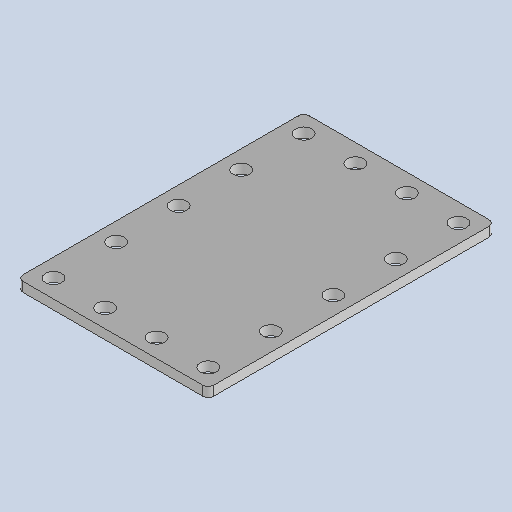
# Autodesk Inventor part: PRS 1607 charging flange rect_940
Saved by Autodesk Inventor 2026.2 (Build 302298000, 298)
## iProperties
Created: 2025-02-13
Part Number: PRS 1607 charging flange rect_940
Material: Steel
Document SubType Name: Sheet Metal
Designer: admin
Mass: 2466.79 g
Surface Area: 934.137 cm^2
Volume: 314.241 cm^3
Density: 7.85 g/cm^3
Flat Pattern Width: 30 cm
Flat Pattern Length: 20 cm
Flat Pattern Area: 600 cm^2
Sheet Metal Rule: AISI304 4mm Die 32
Sheet Metal Width: 300,000 mm
Sheet Metal Length: 200,000 mm
Sheet Metal Area: 60000,000 mm^2
Appearance: Default
Author: pokla
Autodesk Inventor part; units mm, degrees
ref_plane "YZ Plane" through (0, 0, 0) normal (1, 0, 0) x (0, 1, 0)
ref_plane "XZ Plane" through (0, 0, 0) normal (0, 1, 0) x (-1, 0, 0)
ref_plane "XY Plane" through (0, 0, 0) normal (0, 0, 1) x (1, 0, 0)
sketch "Sketch2" plane through (0, 0, 0) normal (0, 0, 1) x (1, 0, 0)
  line L0 (-50, -100) -> (50, -100)
  line L1 (50, -100) -> (50, 100)
  line L2 (50, 100) -> (-50, 100)
  line L3 (-50, 100) -> (-50, -100)
  line L4 (-50, -100) -> (50, 100) construction
  line L5 (50, -100) -> (-50, 100) construction
  line L6 (-100, -150) -> (100, -150)
  line L7 (100, -150) -> (100, 150)
  line L8 (100, 150) -> (-100, 150)
  line L9 (-100, 150) -> (-100, -150)
  point P0 (0, 0)
  dimension "d29" = 100
  dimension "d30" = 200
  dimension "d31" = 50
  measures "d29" distance of L2.end L1.end
  measures "d30" distance of L1.end L0.end
  measures "d31" distance between parallel lines of L3 L9
extrude "Plate2" add sketch "Sketch2" along normal blind 10 contours L3 L2 L1 L0 | L9 L8 L7 L6
sketch "Sketch5" plane through (0, 0, 10) normal (0, 0, 1) x (1, 0, 0)
  line L0 (100, -150) -> (-100, -150) construction
  line L1 (100, 150) -> (100, -150) construction
  line L2 (-100, 150) -> (100, 150) construction
  line L3 (-100, -150) -> (-100, 150) construction
  line L4 (-81, 131) -> (81, 131) construction
  line L5 (81, 131) -> (81, -131) construction
  line L6 (81, -131) -> (-81, -131) construction
  line L7 (-81, -131) -> (-81, 131) construction
  circle A0 centre (-81, -131) radius 8.5
  circle A1 centre (-81, 131) radius 8.5
  circle A2 centre (-81, 0) radius 8.5
  circle A3 centre (-81, -65.5) radius 8.5
  circle A4 centre (-81, 65.5) radius 8.5
  line L8 (-50, 0) -> (50, 0) construction
  circle A5 centre (-27, -131) radius 8.5
  circle A6 centre (-27, -65.5) radius 8.5
  circle A7 centre (-27, 0) radius 8.5
  circle A8 centre (-27, 65.5) radius 8.5
  circle A9 centre (-27, 131) radius 8.5
  circle A10 centre (27, -131) radius 8.5
  circle A11 centre (27, -65.5) radius 8.5
  circle A12 centre (27, 0) radius 8.5
  circle A13 centre (27, 65.5) radius 8.5
  circle A14 centre (27, 131) radius 8.5
  circle A15 centre (81, -131) radius 8.5
  circle A16 centre (81, -65.5) radius 8.5
  circle A17 centre (81, 0) radius 8.5
  circle A18 centre (81, 65.5) radius 8.5
  circle A19 centre (81, 131) radius 8.5
  point P0 (0, 0)
  point P1 (0, -131)
  dimension "d33" = 17
  dimension "d34" = 19
  dimension "d35" = 65.5
  dimension "d36" = 65.5
  dimension "d39" = 54
  constraints: 20 centre point, 10 end point, 8 coincident, 4 equal radius, 2 midpoint, 2 point on line, 1 horizontal, 40 other
  measures "d33" diameter of A0
  measures "d34" distance between parallel lines of L0 L6
  measures "d35" distance of A3.centre L6.end
  measures "d36" distance of A3.centre A2.centre
  measures "d39" distance of L6.end point (-27, -131)
extrude "Cut3" cut sketch "Sketch5" against normal blind 10 contours A0 | A1 | A2 | A3 | A4 | A5 | A9 | A10 | A14 | A15 | A16 | A17 | A18 | A19
fillet "Corner Round1" radius 6 4 edges at (-100, -150, 5) (-100, 150, 5) (100, 150, 5) (100, -150, 5)
equation "\"d35\" = d36"
equation "\"d44\" = Thickness"
equation "\"d14\" = Thickness"
equation "\"BendReliefDepth\" = 0.5 * Thickness"
equation "\"TransitionRadius\" = BendRadius"
equation "\"JacobiRadiusSize\" = BendRadius"
equation "\"Thickness\" = 10"
equation "\"BendRadius\" = 6"
body "Solid3"
